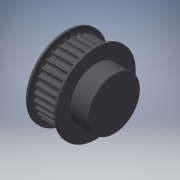
# Autodesk Inventor part: ToothedBeltWheel
Saved by Autodesk Inventor 2018.3 (Build 223284000, 284)
## iProperties
Category: PARTsolutions
Company: MAEDLER
Created: 2018-07-07
Part Number: ToothedBeltWheel
Catalog Web Link: www.cadenas.de
Description: zrr_htd_3m15-HTD Pulleys Profile 3M, Timing Belt Width 15mm
Vendor: MAEDLER
Document SubType Name: Modeling
Designer: psAdmin
Manufacturer: MAEDLER
Mass: 72 g
Surface Area: 81.6114 cm^2
Volume: 25.9232 cm^3
Density: 1 g/cm^3
Material: Allgemein
Appearance: PSOLRGB-175-175-175
PSOL_IDENT_0: {$CADENAS_DATA\23d-libs\maedler\antriebselemente\zahnriemenraeder_zahnriemen\zahnriemenraeder\htd-pr
PSOL_IDENT_1: ofil\zrr_htd_3m15.prj},197 {VTYP=3D},{NB=zrr_htd_3m15_6_17034000},{LINA=zrr_htd_3m15_6_17034000},{NN=
PSOL_IDENT_2: zrr_htd_3m15},{DATE=16.06.2017 10:47:49},{GEOMDATE=09.06.2016 09:07:07},{VERSION=},{LINEID=360},{LIN
PSOL_IDENT_3: ESUBID=-1},{WBVAR=BX}  {NB=zrr_htd_3m15_6_17034000},{LINA=zrr_htd_3m15_6_17034000},{KT=DUMMY},{ARTNR=
PSOL_IDENT_4: 17034000},{PDF=PDF Katalogseite},{AUSF=40-3M-15-1F},{MAT=Aluminium},{ZTL=3.000},{ZRB=15.000},{Z=40.0
PSOL_IDENT_5: 00},{AUS=1F},{ZS=37.440},{BS=42.000},{DO=38.200},{ND=28.000},{B=20.000},{L=30.000},{I=0.000},{VB=6.0
PSOL_IDENT_6: 00},{FB=16.500},{BX=6},{GEW=72.000},{ZT=1.200},{ZB=1.800},{T=1.000},{BB=1.000}
NN: zrr_htd_3m15
NT: HTD-Zahnriemenräder Profil 3M, Zahnriemenbreite 15mm
NB: zrr_htd_3m15_6_17034000
NBSYN: zrr_htd_3m15_$BX._$ARTNR.
LINA: zrr_htd_3m15_6_17034000
ARTNR: 17034000
PDF: PDF Katalogseite
AUSF: 40-3M-15-1F
MAT: Aluminium
ZTL: 3.000
ZRB: 15.000
Z: 40.000
AUS: 1F
ZS: 37.440
BS: 42.000
DO: 38.200
ND: 28.000
B: 20.000
L: 30.000
I: 0.000
VB: 6.000
FB: 16.500
BX: 6
GEW: 72.000
ZT: 1.200
ZB: 1.800
T: 1.000
BB: 1.000
SUPPLIER: MAEDLER
ARTICLENO: zrr_htd_3m15_6_17034000
BOMINFO: zrr_htd_3m15_6_17034000
CREATOR: CADENAS GmbH
Title: zrr_htd_3m15_6_17034000
Author: Cadenas PARTsolutions
Comments: HTD Pulleys Profile 3M, Timing Belt Width 15mm
Autodesk Inventor part; units mm, degrees
ref_plane "YZ Plane" through (0, 0, 0) normal (1, 0, 0) x (0, 1, 0)
ref_plane "XZ Plane" through (0, 0, 0) normal (0, 1, 0) x (-1, 0, 0)
ref_plane "XY Plane" through (0, 0, 0) normal (0, 0, 1) x (1, 0, 0)
sketch "Sketch_3" plane through (0, 0, 0) normal (0, 0, 1) x (1, 0, 0)
  line L0 (20.6, 0) -> (0, 0)
  line L1 (0, 0) -> (0, 17)
  line L2 (0, 17) -> (0.8, 17)
  line L3 (0.8, 17) -> (1.1527, 15)
  line L4 (1.1527, 15) -> (11.6473, 15)
  line L5 (11.6473, 15) -> (12, 17)
  line L6 (12, 17) -> (12.8, 17)
  line L7 (12.8, 17) -> (12.8, 11)
  line L8 (20.6, 0) -> (0, 0)
  line L9 (0, 20.4) -> (0, -3.4) construction
  line L10 (-4.12, 0) -> (24.72, 0) construction
  line L11 (6.4, 15) -> (6.4, 0) construction
  line L12 (12.8, 11) -> (20.6, 11)
  line L13 (20.6, 11) -> (20.6, 0)
  dimension "d5" = 15
  dimension "d6" = 0.8
  dimension "d7" = 2
  dimension "d9" = 100
  dimension "d15" = 12.8
  dimension "d16" = 20.6
  dimension "d17" = 11
  constraints: 24 end point, 4 collinear, 3 point on line, 2 perpendicular, 1 horizontal, 1 midpoint, 1 vertical, 1 other
  measures "d5" distance between parallel lines of L0 L4
  measures "d6" distance of L1.end L2.end
  measures "d7" distance between parallel lines of L4 L6
  measures "d9" angle of L4 L3
  measures "d15" distance between parallel lines of L7 L1
  measures "d16" distance between parallel lines of L13 L1
  measures "d17" distance between parallel lines of L0 L12
revolve "Revolution1" add sketch "Sketch_3" angle 360 about axis through (20.6, 0, 0) along (1, 0, 0)
sketch "Sketch_4" plane through (1, 0, 0) normal (1, 0, 0) x (0, 0, -1)
  circle A0 centre (0, 0) radius 300
  circle A1 centre (0, 0) radius 206
  arc A2 (-14.8517, -1.199) -> (-14.8283, -1.4605) centre (0, 0) ccw
  arc A3 (-14.8283, -1.4605) -> (-14.8002, -1.7214) centre (0, 0) ccw
  arc A4 (-14.3324, -4.0734) -> (-14.8002, -1.7214) centre (-14.6137, -2.9068) ccw
  arc A5 (-14.3324, -4.0734) -> (-14.2584, -4.3252) centre (0, 0) ccw
  arc A6 (-14.2584, -4.3252) -> (-14.18, -4.5757) centre (0, 0) ccw
  arc A7 (-13.2623, -6.7912) -> (-14.18, -4.5757) centre (-13.7658, -5.702) ccw
  arc A8 (-13.2623, -6.7912) -> (-13.1406, -7.0238) centre (0, 0) ccw
  arc A9 (-13.1406, -7.0238) -> (-13.0149, -7.2542) centre (0, 0) ccw
  arc A10 (-11.6826, -9.2481) -> (-13.0149, -7.2542) centre (-12.3889, -8.278) ccw
  arc A11 (-11.6826, -9.2481) -> (-11.5179, -9.4525) centre (0, 0) ccw
  arc A12 (-11.5179, -9.4525) -> (-11.3496, -9.6539) centre (0, 0) ccw
  arc A13 (-9.6539, -11.3496) -> (-11.3496, -9.6539) centre (-10.5359, -10.5359) ccw
  arc A14 (-9.6539, -11.3496) -> (-9.4525, -11.5179) centre (0, 0) ccw
  arc A15 (-9.4525, -11.5179) -> (-9.2481, -11.6826) centre (0, 0) ccw
  arc A16 (-7.2542, -13.0149) -> (-9.2481, -11.6826) centre (-8.278, -12.3889) ccw
  arc A17 (-7.2542, -13.0149) -> (-7.0238, -13.1406) centre (0, 0) ccw
  arc A18 (-7.0238, -13.1406) -> (-6.7912, -13.2623) centre (0, 0) ccw
  arc A19 (-4.5757, -14.18) -> (-6.7912, -13.2623) centre (-5.702, -13.7658) ccw
  arc A20 (-4.5757, -14.18) -> (-4.3252, -14.2584) centre (0, 0) ccw
  arc A21 (-4.3252, -14.2584) -> (-4.0734, -14.3324) centre (0, 0) ccw
  arc A22 (-1.7214, -14.8002) -> (-4.0734, -14.3324) centre (-2.9068, -14.6137) ccw
  arc A23 (-1.7214, -14.8002) -> (-1.4605, -14.8283) centre (0, 0) ccw
  arc A24 (-1.4605, -14.8283) -> (-1.199, -14.8517) centre (0, 0) ccw
  arc A25 (1.199, -14.8517) -> (-1.199, -14.8517) centre (0, -14.9) ccw
  arc A26 (1.199, -14.8517) -> (1.4605, -14.8283) centre (0, 0) ccw
  arc A27 (1.4605, -14.8283) -> (1.7214, -14.8002) centre (0, 0) ccw
  arc A28 (4.0734, -14.3324) -> (1.7214, -14.8002) centre (2.9068, -14.6137) ccw
  arc A29 (4.0734, -14.3324) -> (4.3252, -14.2584) centre (0, 0) ccw
  arc A30 (4.3252, -14.2584) -> (4.5757, -14.18) centre (0, 0) ccw
  arc A31 (6.7912, -13.2623) -> (4.5757, -14.18) centre (5.702, -13.7658) ccw
  arc A32 (6.7912, -13.2623) -> (7.0238, -13.1406) centre (0, 0) ccw
  arc A33 (7.0238, -13.1406) -> (7.2542, -13.0149) centre (0, 0) ccw
  arc A34 (9.2481, -11.6826) -> (7.2542, -13.0149) centre (8.278, -12.3889) ccw
  arc A35 (9.2481, -11.6826) -> (9.4525, -11.5179) centre (0, 0) ccw
  arc A36 (9.4525, -11.5179) -> (9.6539, -11.3496) centre (0, 0) ccw
  arc A37 (11.3496, -9.6539) -> (9.6539, -11.3496) centre (10.5359, -10.5359) ccw
  arc A38 (11.3496, -9.6539) -> (11.5179, -9.4525) centre (0, 0) ccw
  arc A39 (11.5179, -9.4525) -> (11.6826, -9.2481) centre (0, 0) ccw
  arc A40 (13.0149, -7.2542) -> (11.6826, -9.2481) centre (12.3889, -8.278) ccw
  arc A41 (13.0149, -7.2542) -> (13.1406, -7.0238) centre (0, 0) ccw
  arc A42 (13.1406, -7.0238) -> (13.2623, -6.7912) centre (0, 0) ccw
  arc A43 (14.18, -4.5757) -> (13.2623, -6.7912) centre (13.7658, -5.702) ccw
  arc A44 (14.18, -4.5757) -> (14.2584, -4.3252) centre (0, 0) ccw
  arc A45 (14.2584, -4.3252) -> (14.3324, -4.0734) centre (0, 0) ccw
  arc A46 (14.8002, -1.7214) -> (14.3324, -4.0734) centre (14.6137, -2.9068) ccw
  arc A47 (14.8002, -1.7214) -> (14.8283, -1.4605) centre (0, 0) ccw
  arc A48 (14.8283, -1.4605) -> (14.8517, -1.199) centre (0, 0) ccw
  arc A49 (14.8517, 1.199) -> (14.8517, -1.199) centre (14.9, 0) ccw
  arc A50 (14.8517, 1.199) -> (14.8283, 1.4605) centre (0, 0) ccw
  arc A51 (14.8283, 1.4605) -> (14.8002, 1.7214) centre (0, 0) ccw
  arc A52 (14.3324, 4.0734) -> (14.8002, 1.7214) centre (14.6137, 2.9068) ccw
  arc A53 (14.3324, 4.0734) -> (14.2584, 4.3252) centre (0, 0) ccw
  arc A54 (14.2584, 4.3252) -> (14.18, 4.5757) centre (0, 0) ccw
  arc A55 (13.2623, 6.7912) -> (14.18, 4.5757) centre (13.7658, 5.702) ccw
  arc A56 (13.2623, 6.7912) -> (13.1406, 7.0238) centre (0, 0) ccw
  arc A57 (13.1406, 7.0238) -> (13.0149, 7.2542) centre (0, 0) ccw
  arc A58 (11.6826, 9.2481) -> (13.0149, 7.2542) centre (12.3889, 8.278) ccw
  arc A59 (11.6826, 9.2481) -> (11.5179, 9.4525) centre (0, 0) ccw
  arc A60 (11.5179, 9.4525) -> (11.3496, 9.6539) centre (0, 0) ccw
  arc A61 (9.6539, 11.3496) -> (11.3496, 9.6539) centre (10.5359, 10.5359) ccw
  arc A62 (9.6539, 11.3496) -> (9.4525, 11.5179) centre (0, 0) ccw
  arc A63 (9.4525, 11.5179) -> (9.2481, 11.6826) centre (0, 0) ccw
  arc A64 (7.2542, 13.0149) -> (9.2481, 11.6826) centre (8.278, 12.3889) ccw
  arc A65 (7.2542, 13.0149) -> (7.0238, 13.1406) centre (0, 0) ccw
  arc A66 (7.0238, 13.1406) -> (6.7912, 13.2623) centre (0, 0) ccw
  arc A67 (4.5757, 14.18) -> (6.7912, 13.2623) centre (5.702, 13.7658) ccw
  arc A68 (4.5757, 14.18) -> (4.3252, 14.2584) centre (0, 0) ccw
  arc A69 (4.3252, 14.2584) -> (4.0734, 14.3324) centre (0, 0) ccw
  arc A70 (1.7214, 14.8002) -> (4.0734, 14.3324) centre (2.9068, 14.6137) ccw
  arc A71 (1.7214, 14.8002) -> (1.4605, 14.8283) centre (0, 0) ccw
  arc A72 (1.4605, 14.8283) -> (1.199, 14.8517) centre (0, 0) ccw
  arc A73 (-1.199, 14.8517) -> (1.199, 14.8517) centre (0, 14.9) ccw
  arc A74 (-1.199, 14.8517) -> (-1.4605, 14.8283) centre (0, 0) ccw
  arc A75 (-1.4605, 14.8283) -> (-1.7214, 14.8002) centre (0, 0) ccw
  arc A76 (-4.0734, 14.3324) -> (-1.7214, 14.8002) centre (-2.9068, 14.6137) ccw
  arc A77 (-4.0734, 14.3324) -> (-4.3252, 14.2584) centre (0, 0) ccw
  arc A78 (-4.3252, 14.2584) -> (-4.5757, 14.18) centre (0, 0) ccw
  arc A79 (-6.7912, 13.2623) -> (-4.5757, 14.18) centre (-5.702, 13.7658) ccw
  arc A80 (-6.7912, 13.2623) -> (-7.0238, 13.1406) centre (0, 0) ccw
  arc A81 (-7.0238, 13.1406) -> (-7.2542, 13.0149) centre (0, 0) ccw
  arc A82 (-9.2481, 11.6826) -> (-7.2542, 13.0149) centre (-8.278, 12.3889) ccw
  arc A83 (-9.2481, 11.6826) -> (-9.4525, 11.5179) centre (0, 0) ccw
  arc A84 (-9.4525, 11.5179) -> (-9.6539, 11.3496) centre (0, 0) ccw
  arc A85 (-11.3496, 9.6539) -> (-9.6539, 11.3496) centre (-10.5359, 10.5359) ccw
  arc A86 (-11.3496, 9.6539) -> (-11.5179, 9.4525) centre (0, 0) ccw
  arc A87 (-11.5179, 9.4525) -> (-11.6826, 9.2481) centre (0, 0) ccw
  arc A88 (-13.0149, 7.2542) -> (-11.6826, 9.2481) centre (-12.3889, 8.278) ccw
  arc A89 (-13.0149, 7.2542) -> (-13.1406, 7.0238) centre (0, 0) ccw
  arc A90 (-13.1406, 7.0238) -> (-13.2623, 6.7912) centre (0, 0) ccw
  arc A91 (-14.18, 4.5757) -> (-13.2623, 6.7912) centre (-13.7658, 5.702) ccw
  arc A92 (-14.18, 4.5757) -> (-14.2584, 4.3252) centre (0, 0) ccw
  arc A93 (-14.2584, 4.3252) -> (-14.3324, 4.0734) centre (0, 0) ccw
  arc A94 (-14.8002, 1.7214) -> (-14.3324, 4.0734) centre (-14.6137, 2.9068) ccw
  arc A95 (-14.8002, 1.7214) -> (-14.8283, 1.4605) centre (0, 0) ccw
  arc A96 (-14.8283, 1.4605) -> (-14.8517, 1.199) centre (0, 0) ccw
  arc A97 (-14.8517, -1.199) -> (-14.8517, 1.199) centre (-14.9, 0) ccw
  line L0 (0.2687, 0) -> (-14.9, 0) construction
  line L1 (0, 0) -> (-14.6137, 2.9068) construction
  dimension "d11" = 11.25
  constraints: 192 point on circle, 98 centre point, 4 end point, 1 coincident, 1 horizontal
  measures "d11" angle of L0 L1
extrude "Extrusion1" cut sketch "Sketch_4" along normal blind 11 contours A1
sketch "Sketch_9_ALT_Drilling_1" plane through (0, 0, 0) normal (1, 0, 0) x (0, 1, 0)
  circle A0 centre (0, 0) radius 2
  line L0 (0, -2.8) -> (0, 2.8) construction
  line L1 (-2.8, 0) -> (2.8, 0) construction
  dimension "d10" = 4
  constraints: 1 centre point, 1 coincident
  measures "d10" diameter of A0
body "Solid1"
